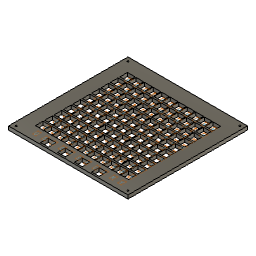
Wordclock (Autodesk Fusion 360 design; units mm, degrees)
Autodesk Fusion 360 part; units mm, degrees
(part 1 of 9)
sketch "Sketch1" plane through (0, 0, 0) normal (0, 0, 1) x (1, 0, 0)
  line L0 (117.5, 117.5) -> (-117.5, 117.5)
  line L1 (-117.5, 117.5) -> (-117.5, -117.5)
  line L2 (-117.5, -117.5) -> (117.5, -117.5)
  line L3 (117.5, -117.5) -> (117.5, 117.5)
  line L4 (117.5, 117.5) -> (-117.5, -117.5) construction
  line L5 (-117.5, 117.5) -> (117.5, -117.5) construction
  circle A0 centre (-110, 110) radius 1.6
  circle A1 centre (110, 110) radius 1.6
  circle A2 centre (-110, -110) radius 1.6
  circle A3 centre (110, -110) radius 1.6
  line L6 (-91.5, 90.5) -> (-76.5, 90.5)
  line L7 (-76.5, 90.5) -> (-76.5, 75.5)
  line L8 (-76.5, 75.5) -> (-91.5, 75.5)
  line L9 (-91.5, 75.5) -> (-91.5, 90.5)
  line L10 (-59.7, 75.5) -> (-74.7, 75.5)
  line L11 (-74.7, 75.5) -> (-74.7, 90.5)
  line L12 (-74.7, 90.5) -> (-59.7, 90.5)
  line L13 (-59.7, 90.5) -> (-59.7, 75.5)
  line L14 (-42.9, 75.5) -> (-57.9, 75.5)
  line L15 (-57.9, 75.5) -> (-57.9, 90.5)
  line L16 (-57.9, 90.5) -> (-42.9, 90.5)
  line L17 (-42.9, 90.5) -> (-42.9, 75.5)
  line L18 (-26.1, 75.5) -> (-41.1, 75.5)
  line L19 (-41.1, 75.5) -> (-41.1, 90.5)
  line L20 (-41.1, 90.5) -> (-26.1, 90.5)
  line L21 (-26.1, 90.5) -> (-26.1, 75.5)
  line L22 (-9.3, 75.5) -> (-24.3, 75.5)
  line L23 (-24.3, 75.5) -> (-24.3, 90.5)
  line L24 (-24.3, 90.5) -> (-9.3, 90.5)
  line L25 (-9.3, 90.5) -> (-9.3, 75.5)
  line L26 (7.5, 75.5) -> (-7.5, 75.5)
  line L27 (-7.5, 75.5) -> (-7.5, 90.5)
  line L28 (-7.5, 90.5) -> (7.5, 90.5)
  line L29 (7.5, 90.5) -> (7.5, 75.5)
  line L30 (24.3, 75.5) -> (9.3, 75.5)
  line L31 (9.3, 75.5) -> (9.3, 90.5)
  line L32 (9.3, 90.5) -> (24.3, 90.5)
  line L33 (24.3, 90.5) -> (24.3, 75.5)
  line L34 (41.1, 75.5) -> (26.1, 75.5)
  line L35 (26.1, 75.5) -> (26.1, 90.5)
  line L36 (26.1, 90.5) -> (41.1, 90.5)
  line L37 (41.1, 90.5) -> (41.1, 75.5)
  line L38 (57.9, 75.5) -> (42.9, 75.5)
  line L39 (42.9, 75.5) -> (42.9, 90.5)
  line L40 (42.9, 90.5) -> (57.9, 90.5)
  line L41 (57.9, 90.5) -> (57.9, 75.5)
  line L42 (74.7, 75.5) -> (59.7, 75.5)
  line L43 (59.7, 75.5) -> (59.7, 90.5)
  line L44 (59.7, 90.5) -> (74.7, 90.5)
  line L45 (74.7, 90.5) -> (74.7, 75.5)
  line L46 (91.5, 75.5) -> (76.5, 75.5)
  line L47 (76.5, 75.5) -> (76.5, 90.5)
  line L48 (76.5, 90.5) -> (91.5, 90.5)
  line L49 (91.5, 90.5) -> (91.5, 75.5)
  line L50 (-76.5, 57.055) -> (-91.5, 57.055)
  line L51 (-91.5, 57.055) -> (-91.5, 72.055)
  line L52 (-91.5, 72.055) -> (-76.5, 72.055)
  line L53 (-76.5, 72.055) -> (-76.5, 57.055)
  line L54 (-59.7, 57.055) -> (-74.7, 57.055)
  line L55 (-74.7, 57.055) -> (-74.7, 72.055)
  line L56 (-74.7, 72.055) -> (-59.7, 72.055)
  line L57 (-59.7, 72.055) -> (-59.7, 57.055)
  line L58 (-42.9, 57.055) -> (-57.9, 57.055)
  line L59 (-57.9, 57.055) -> (-57.9, 72.055)
  line L60 (-57.9, 72.055) -> (-42.9, 72.055)
  line L61 (-42.9, 72.055) -> (-42.9, 57.055)
  line L62 (-26.1, 57.055) -> (-41.1, 57.055)
  line L63 (-41.1, 57.055) -> (-41.1, 72.055)
  line L64 (-41.1, 72.055) -> (-26.1, 72.055)
  line L65 (-26.1, 72.055) -> (-26.1, 57.055)
  line L66 (-9.3, 57.055) -> (-24.3, 57.055)
  line L67 (-24.3, 57.055) -> (-24.3, 72.055)
  line L68 (-24.3, 72.055) -> (-9.3, 72.055)
  line L69 (-9.3, 72.055) -> (-9.3, 57.055)
  line L70 (7.5, 57.055) -> (-7.5, 57.055)
  line L71 (-7.5, 57.055) -> (-7.5, 72.055)
  line L72 (-7.5, 72.055) -> (7.5, 72.055)
  line L73 (7.5, 72.055) -> (7.5, 57.055)
  line L74 (24.3, 57.055) -> (9.3, 57.055)
  line L75 (9.3, 57.055) -> (9.3, 72.055)
  line L76 (9.3, 72.055) -> (24.3, 72.055)
  line L77 (24.3, 72.055) -> (24.3, 57.055)
  line L78 (41.1, 57.055) -> (26.1, 57.055)
  line L79 (26.1, 57.055) -> (26.1, 72.055)
  line L80 (26.1, 72.055) -> (41.1, 72.055)
  line L81 (41.1, 72.055) -> (41.1, 57.055)
  line L82 (57.9, 57.055) -> (42.9, 57.055)
  line L83 (42.9, 57.055) -> (42.9, 72.055)
  line L84 (42.9, 72.055) -> (57.9, 72.055)
  line L85 (57.9, 72.055) -> (57.9, 57.055)
  line L86 (74.7, 57.055) -> (59.7, 57.055)
  line L87 (59.7, 57.055) -> (59.7, 72.055)
  line L88 (59.7, 72.055) -> (74.7, 72.055)
  line L89 (74.7, 72.055) -> (74.7, 57.055)
  line L90 (91.5, 57.055) -> (76.5, 57.055)
  line L91 (76.5, 57.055) -> (76.5, 72.055)
  line L92 (76.5, 72.055) -> (91.5, 72.055)
  line L93 (91.5, 72.055) -> (91.5, 57.055)
  line L94 (-76.5, 38.61) -> (-91.5, 38.61)
  line L95 (-91.5, 38.61) -> (-91.5, 53.61)
  line L96 (-91.5, 53.61) -> (-76.5, 53.61)
  line L97 (-76.5, 53.61) -> (-76.5, 38.61)
  line L98 (-59.7, 38.61) -> (-74.7, 38.61)
  line L99 (-74.7, 38.61) -> (-74.7, 53.61)
  line L100 (-74.7, 53.61) -> (-59.7, 53.61)
  line L101 (-59.7, 53.61) -> (-59.7, 38.61)
  line L102 (-42.9, 38.61) -> (-57.9, 38.61)
  line L103 (-57.9, 38.61) -> (-57.9, 53.61)
  line L104 (-57.9, 53.61) -> (-42.9, 53.61)
  line L105 (-42.9, 53.61) -> (-42.9, 38.61)
  line L106 (-26.1, 38.61) -> (-41.1, 38.61)
  line L107 (-41.1, 38.61) -> (-41.1, 53.61)
  line L108 (-41.1, 53.61) -> (-26.1, 53.61)
  line L109 (-26.1, 53.61) -> (-26.1, 38.61)
  line L110 (-9.3, 38.61) -> (-24.3, 38.61)
  line L111 (-24.3, 38.61) -> (-24.3, 53.61)
  line L112 (-24.3, 53.61) -> (-9.3, 53.61)
  line L113 (-9.3, 53.61) -> (-9.3, 38.61)
  line L114 (7.5, 38.61) -> (-7.5, 38.61)
  line L115 (-7.5, 38.61) -> (-7.5, 53.61)
  line L116 (-7.5, 53.61) -> (7.5, 53.61)
  line L117 (7.5, 53.61) -> (7.5, 38.61)
  line L118 (24.3, 38.61) -> (9.3, 38.61)
  line L119 (9.3, 38.61) -> (9.3, 53.61)
  line L120 (9.3, 53.61) -> (24.3, 53.61)
  line L121 (24.3, 53.61) -> (24.3, 38.61)
  line L122 (41.1, 38.61) -> (26.1, 38.61)
  line L123 (26.1, 38.61) -> (26.1, 53.61)
  line L124 (26.1, 53.61) -> (41.1, 53.61)
  line L125 (41.1, 53.61) -> (41.1, 38.61)
  line L126 (57.9, 38.61) -> (42.9, 38.61)
  line L127 (42.9, 38.61) -> (42.9, 53.61)
  line L128 (42.9, 53.61) -> (57.9, 53.61)
  line L129 (57.9, 53.61) -> (57.9, 38.61)
  line L130 (74.7, 38.61) -> (59.7, 38.61)
  line L131 (59.7, 38.61) -> (59.7, 53.61)
  line L132 (59.7, 53.61) -> (74.7, 53.61)
  line L133 (74.7, 53.61) -> (74.7, 38.61)
  line L134 (91.5, 38.61) -> (76.5, 38.61)
  line L135 (76.5, 38.61) -> (76.5, 53.61)
  line L136 (76.5, 53.61) -> (91.5, 53.61)
  line L137 (91.5, 53.61) -> (91.5, 38.61)
  line L138 (-76.5, 20.165) -> (-91.5, 20.165)
  line L139 (-91.5, 20.165) -> (-91.5, 35.165)
  line L140 (-91.5, 35.165) -> (-76.5, 35.165)
  line L141 (-76.5, 35.165) -> (-76.5, 20.165)
  line L142 (-59.7, 20.165) -> (-74.7, 20.165)
  line L143 (-74.7, 20.165) -> (-74.7, 35.165)
  line L144 (-74.7, 35.165) -> (-59.7, 35.165)
  line L145 (-59.7, 35.165) -> (-59.7, 20.165)
  line L146 (-42.9, 20.165) -> (-57.9, 20.165)
  line L147 (-57.9, 20.165) -> (-57.9, 35.165)
  line L148 (-57.9, 35.165) -> (-42.9, 35.165)
  line L149 (-42.9, 35.165) -> (-42.9, 20.165)
  line L150 (-26.1, 20.165) -> (-41.1, 20.165)
  line L151 (-41.1, 20.165) -> (-41.1, 35.165)
  line L152 (-41.1, 35.165) -> (-26.1, 35.165)
  line L153 (-26.1, 35.165) -> (-26.1, 20.165)
  line L154 (-9.3, 20.165) -> (-24.3, 20.165)
  line L155 (-24.3, 20.165) -> (-24.3, 35.165)
  line L156 (-24.3, 35.165) -> (-9.3, 35.165)
  line L157 (-9.3, 35.165) -> (-9.3, 20.165)
  line L158 (7.5, 20.165) -> (-7.5, 20.165)
  line L159 (-7.5, 20.165) -> (-7.5, 35.165)
  line L160 (-7.5, 35.165) -> (7.5, 35.165)
  line L161 (7.5, 35.165) -> (7.5, 20.165)
  line L162 (24.3, 20.165) -> (9.3, 20.165)
  line L163 (9.3, 20.165) -> (9.3, 35.165)
  line L164 (9.3, 35.165) -> (24.3, 35.165)
  line L165 (24.3, 35.165) -> (24.3, 20.165)
  line L166 (41.1, 20.165) -> (26.1, 20.165)
  line L167 (26.1, 20.165) -> (26.1, 35.165)
  line L168 (26.1, 35.165) -> (41.1, 35.165)
  line L169 (41.1, 35.165) -> (41.1, 20.165)
  line L170 (57.9, 20.165) -> (42.9, 20.165)
  line L171 (42.9, 20.165) -> (42.9, 35.165)
  line L172 (42.9, 35.165) -> (57.9, 35.165)
  line L173 (57.9, 35.165) -> (57.9, 20.165)
  line L174 (74.7, 20.165) -> (59.7, 20.165)
  line L175 (59.7, 20.165) -> (59.7, 35.165)
  line L176 (59.7, 35.165) -> (74.7, 35.165)
  line L177 (74.7, 35.165) -> (74.7, 20.165)
  line L178 (91.5, 20.165) -> (76.5, 20.165)
  line L179 (76.5, 20.165) -> (76.5, 35.165)
  line L180 (76.5, 35.165) -> (91.5, 35.165)
  line L181 (91.5, 35.165) -> (91.5, 20.165)
  line L182 (-76.5, 1.72) -> (-91.5, 1.72)
  line L183 (-91.5, 1.72) -> (-91.5, 16.72)
  line L184 (-91.5, 16.72) -> (-76.5, 16.72)
  line L185 (-76.5, 16.72) -> (-76.5, 1.72)
  line L186 (-59.7, 1.72) -> (-74.7, 1.72)
  line L187 (-74.7, 1.72) -> (-74.7, 16.72)
  line L188 (-74.7, 16.72) -> (-59.7, 16.72)
  line L189 (-59.7, 16.72) -> (-59.7, 1.72)
  line L190 (-42.9, 1.72) -> (-57.9, 1.72)
  line L191 (-57.9, 1.72) -> (-57.9, 16.72)
  line L192 (-57.9, 16.72) -> (-42.9, 16.72)
  line L193 (-42.9, 16.72) -> (-42.9, 1.72)
  line L194 (-26.1, 1.72) -> (-41.1, 1.72)
  line L195 (-41.1, 1.72) -> (-41.1, 16.72)
  line L196 (-41.1, 16.72) -> (-26.1, 16.72)
  line L197 (-26.1, 16.72) -> (-26.1, 1.72)
  line L198 (-9.3, 1.72) -> (-24.3, 1.72)
  line L199 (-24.3, 1.72) -> (-24.3, 16.72)
  line L200 (-24.3, 16.72) -> (-9.3, 16.72)
  line L201 (-9.3, 16.72) -> (-9.3, 1.72)
  line L202 (7.5, 1.72) -> (-7.5, 1.72)
  line L203 (-7.5, 1.72) -> (-7.5, 16.72)
  line L204 (-7.5, 16.72) -> (7.5, 16.72)
  line L205 (7.5, 16.72) -> (7.5, 1.72)
  line L206 (24.3, 1.72) -> (9.3, 1.72)
  line L207 (9.3, 1.72) -> (9.3, 16.72)
  line L208 (9.3, 16.72) -> (24.3, 16.72)
  line L209 (24.3, 16.72) -> (24.3, 1.72)
  line L210 (41.1, 1.72) -> (26.1, 1.72)
  line L211 (26.1, 1.72) -> (26.1, 16.72)
  line L212 (26.1, 16.72) -> (41.1, 16.72)
  line L213 (41.1, 16.72) -> (41.1, 1.72)
  line L214 (57.9, 1.72) -> (42.9, 1.72)
  line L215 (42.9, 1.72) -> (42.9, 16.72)
  line L216 (42.9, 16.72) -> (57.9, 16.72)
  line L217 (57.9, 16.72) -> (57.9, 1.72)
  line L218 (74.7, 1.72) -> (59.7, 1.72)
  line L219 (59.7, 1.72) -> (59.7, 16.72)
  line L220 (59.7, 16.72) -> (74.7, 16.72)
  line L221 (74.7, 16.72) -> (74.7, 1.72)
  line L222 (91.5, 1.72) -> (76.5, 1.72)
  line L223 (76.5, 1.72) -> (76.5, 16.72)
  line L224 (76.5, 16.72) -> (91.5, 16.72)
  line L225 (91.5, 16.72) -> (91.5, 1.72)
  line L226 (-76.5, -16.725) -> (-91.5, -16.725)
  line L227 (-91.5, -16.725) -> (-91.5, -1.725)
  line L228 (-91.5, -1.725) -> (-76.5, -1.725)
  line L229 (-76.5, -1.725) -> (-76.5, -16.725)
  line L230 (-59.7, -16.725) -> (-74.7, -16.725)
  line L231 (-74.7, -16.725) -> (-74.7, -1.725)
  line L232 (-74.7, -1.725) -> (-59.7, -1.725)
  line L233 (-59.7, -1.725) -> (-59.7, -16.725)
  line L234 (-42.9, -16.725) -> (-57.9, -16.725)
  line L235 (-57.9, -16.725) -> (-57.9, -1.725)
  line L236 (-57.9, -1.725) -> (-42.9, -1.725)
  line L237 (-42.9, -1.725) -> (-42.9, -16.725)
  line L238 (-26.1, -16.725) -> (-41.1, -16.725)
  line L239 (-41.1, -16.725) -> (-41.1, -1.725)
  line L240 (-41.1, -1.725) -> (-26.1, -1.725)
  line L241 (-26.1, -1.725) -> (-26.1, -16.725)
  line L242 (-9.3, -16.725) -> (-24.3, -16.725)
  line L243 (-24.3, -16.725) -> (-24.3, -1.725)
  line L244 (-24.3, -1.725) -> (-9.3, -1.725)
  line L245 (-9.3, -1.725) -> (-9.3, -16.725)
  line L246 (7.5, -16.725) -> (-7.5, -16.725)
  line L247 (-7.5, -16.725) -> (-7.5, -1.725)
  line L248 (-7.5, -1.725) -> (7.5, -1.725)
  line L249 (7.5, -1.725) -> (7.5, -16.725)
  line L250 (24.3, -16.725) -> (9.3, -16.725)
  line L251 (9.3, -16.725) -> (9.3, -1.725)
  line L252 (9.3, -1.725) -> (24.3, -1.725)
  line L253 (24.3, -1.725) -> (24.3, -16.725)
  line L254 (41.1, -16.725) -> (26.1, -16.725)
  line L255 (26.1, -16.725) -> (26.1, -1.725)
  line L256 (26.1, -1.725) -> (41.1, -1.725)
  line L257 (41.1, -1.725) -> (41.1, -16.725)
  line L258 (57.9, -16.725) -> (42.9, -16.725)
  line L259 (42.9, -16.725) -> (42.9, -1.725)
  line L260 (42.9, -1.725) -> (57.9, -1.725)
  line L261 (57.9, -1.725) -> (57.9, -16.725)
  line L262 (74.7, -16.725) -> (59.7, -16.725)
  line L263 (59.7, -16.725) -> (59.7, -1.725)
  line L264 (59.7, -1.725) -> (74.7, -1.725)
  line L265 (74.7, -1.725) -> (74.7, -16.725)
  line L266 (91.5, -16.725) -> (76.5, -16.725)
  line L267 (76.5, -16.725) -> (76.5, -1.725)
  line L268 (76.5, -1.725) -> (91.5, -1.725)
  line L269 (91.5, -1.725) -> (91.5, -16.725)
  line L270 (-76.5, -35.17) -> (-91.5, -35.17)
  line L271 (-91.5, -35.17) -> (-91.5, -20.17)
  line L272 (-91.5, -20.17) -> (-76.5, -20.17)
  line L273 (-76.5, -20.17) -> (-76.5, -35.17)
  line L274 (-59.7, -35.17) -> (-74.7, -35.17)
  line L275 (-74.7, -35.17) -> (-74.7, -20.17)
  line L276 (-74.7, -20.17) -> (-59.7, -20.17)
  line L277 (-59.7, -20.17) -> (-59.7, -35.17)
  line L278 (-42.9, -35.17) -> (-57.9, -35.17)
  line L279 (-57.9, -35.17) -> (-57.9, -20.17)
  line L280 (-57.9, -20.17) -> (-42.9, -20.17)
  line L281 (-42.9, -20.17) -> (-42.9, -35.17)
  line L282 (-26.1, -35.17) -> (-41.1, -35.17)
  line L283 (-41.1, -35.17) -> (-41.1, -20.17)
  line L284 (-41.1, -20.17) -> (-26.1, -20.17)
  line L285 (-26.1, -20.17) -> (-26.1, -35.17)
  line L286 (-9.3, -35.17) -> (-24.3, -35.17)
  line L287 (-24.3, -35.17) -> (-24.3, -20.17)
  line L288 (-24.3, -20.17) -> (-9.3, -20.17)
  line L289 (-9.3, -20.17) -> (-9.3, -35.17)
  line L290 (7.5, -35.17) -> (-7.5, -35.17)
  line L291 (-7.5, -35.17) -> (-7.5, -20.17)
  line L292 (-7.5, -20.17) -> (7.5, -20.17)
  line L293 (7.5, -20.17) -> (7.5, -35.17)
  line L294 (24.3, -35.17) -> (9.3, -35.17)
  line L295 (9.3, -35.17) -> (9.3, -20.17)
  line L296 (9.3, -20.17) -> (24.3, -20.17)
  line L297 (24.3, -20.17) -> (24.3, -35.17)
  line L298 (41.1, -35.17) -> (26.1, -35.17)
  line L299 (26.1, -35.17) -> (26.1, -20.17)
  line L300 (26.1, -20.17) -> (41.1, -20.17)
  line L301 (41.1, -20.17) -> (41.1, -35.17)
  line L302 (57.9, -35.17) -> (42.9, -35.17)
  line L303 (42.9, -35.17) -> (42.9, -20.17)
  line L304 (42.9, -20.17) -> (57.9, -20.17)
  line L305 (57.9, -20.17) -> (57.9, -35.17)
  line L306 (74.7, -35.17) -> (59.7, -35.17)
  line L307 (59.7, -35.17) -> (59.7, -20.17)
  line L308 (59.7, -20.17) -> (74.7, -20.17)
  line L309 (74.7, -20.17) -> (74.7, -35.17)
  line L310 (91.5, -35.17) -> (76.5, -35.17)
  line L311 (76.5, -35.17) -> (76.5, -20.17)
  line L312 (76.5, -20.17) -> (91.5, -20.17)
  line L313 (91.5, -20.17) -> (91.5, -35.17)
  line L314 (-76.5, -53.615) -> (-91.5, -53.615)
  line L315 (-91.5, -53.615) -> (-91.5, -38.615)
  line L316 (-91.5, -38.615) -> (-76.5, -38.615)
  line L317 (-76.5, -38.615) -> (-76.5, -53.615)
  line L318 (-59.7, -53.615) -> (-74.7, -53.615)
  line L319 (-74.7, -53.615) -> (-74.7, -38.615)
  line L320 (-74.7, -38.615) -> (-59.7, -38.615)
  line L321 (-59.7, -38.615) -> (-59.7, -53.615)
  line L322 (-42.9, -53.615) -> (-57.9, -53.615)
  line L323 (-57.9, -53.615) -> (-57.9, -38.615)
  line L324 (-57.9, -38.615) -> (-42.9, -38.615)
  line L325 (-42.9, -38.615) -> (-42.9, -53.615)
  line L326 (-26.1, -53.615) -> (-41.1, -53.615)
  line L327 (-41.1, -53.615) -> (-41.1, -38.615)
  line L328 (-41.1, -38.615) -> (-26.1, -38.615)
  line L329 (-26.1, -38.615) -> (-26.1, -53.615)
  line L330 (-9.3, -53.615) -> (-24.3, -53.615)
  line L331 (-24.3, -53.615) -> (-24.3, -38.615)
  line L332 (-24.3, -38.615) -> (-9.3, -38.615)
  line L333 (-9.3, -38.615) -> (-9.3, -53.615)
  line L334 (7.5, -53.615) -> (-7.5, -53.615)
  line L335 (-7.5, -53.615) -> (-7.5, -38.615)
  line L336 (-7.5, -38.615) -> (7.5, -38.615)
  line L337 (7.5, -38.615) -> (7.5, -53.615)
  line L338 (24.3, -53.615) -> (9.3, -53.615)
  line L339 (9.3, -53.615) -> (9.3, -38.615)
  line L340 (9.3, -38.615) -> (24.3, -38.615)
  line L341 (24.3, -38.615) -> (24.3, -53.615)
  line L342 (41.1, -53.615) -> (26.1, -53.615)
  line L343 (26.1, -53.615) -> (26.1, -38.615)
  line L344 (26.1, -38.615) -> (41.1, -38.615)
  line L345 (41.1, -38.615) -> (41.1, -53.615)
  line L346 (57.9, -53.615) -> (42.9, -53.615)
  line L347 (42.9, -53.615) -> (42.9, -38.615)
  line L348 (42.9, -38.615) -> (57.9, -38.615)
  line L349 (57.9, -38.615) -> (57.9, -53.615)
  line L350 (74.7, -53.615) -> (59.7, -53.615)
  line L351 (59.7, -53.615) -> (59.7, -38.615)
  line L352 (59.7, -38.615) -> (74.7, -38.615)
  line L353 (74.7, -38.615) -> (74.7, -53.615)
  line L354 (91.5, -53.615) -> (76.5, -53.615)
  line L355 (76.5, -53.615) -> (76.5, -38.615)
  line L356 (76.5, -38.615) -> (91.5, -38.615)
  line L357 (91.5, -38.615) -> (91.5, -53.615)
  line L358 (-76.5, -72.06) -> (-91.5, -72.06)
  line L359 (-91.5, -72.06) -> (-91.5, -57.06)
  line L360 (-91.5, -57.06) -> (-76.5, -57.06)
  line L361 (-76.5, -57.06) -> (-76.5, -72.06)
  line L362 (-59.7, -72.06) -> (-74.7, -72.06)
  line L363 (-74.7, -72.06) -> (-74.7, -57.06)
  line L364 (-74.7, -57.06) -> (-59.7, -57.06)
  line L365 (-59.7, -57.06) -> (-59.7, -72.06)
  line L366 (-42.9, -72.06) -> (-57.9, -72.06)
  line L367 (-57.9, -72.06) -> (-57.9, -57.06)
  line L368 (-57.9, -57.06) -> (-42.9, -57.06)
  line L369 (-42.9, -57.06) -> (-42.9, -72.06)
  line L370 (-26.1, -72.06) -> (-41.1, -72.06)
  line L371 (-41.1, -72.06) -> (-41.1, -57.06)
  line L372 (-41.1, -57.06) -> (-26.1, -57.06)
  line L373 (-26.1, -57.06) -> (-26.1, -72.06)
  line L374 (-9.3, -72.06) -> (-24.3, -72.06)
  line L375 (-24.3, -72.06) -> (-24.3, -57.06)
  line L376 (-24.3, -57.06) -> (-9.3, -57.06)
  line L377 (-9.3, -57.06) -> (-9.3, -72.06)
  line L378 (7.5, -72.06) -> (-7.5, -72.06)
  line L379 (-7.5, -72.06) -> (-7.5, -57.06)
  line L380 (-7.5, -57.06) -> (7.5, -57.06)
  line L381 (7.5, -57.06) -> (7.5, -72.06)
  line L382 (24.3, -72.06) -> (9.3, -72.06)
  line L383 (9.3, -72.06) -> (9.3, -57.06)
  line L384 (9.3, -57.06) -> (24.3, -57.06)
  line L385 (24.3, -57.06) -> (24.3, -72.06)
  line L386 (41.1, -72.06) -> (26.1, -72.06)
  line L387 (26.1, -72.06) -> (26.1, -57.06)
  line L388 (26.1, -57.06) -> (41.1, -57.06)
  line L389 (41.1, -57.06) -> (41.1, -72.06)
  line L390 (57.9, -72.06) -> (42.9, -72.06)
  line L391 (42.9, -72.06) -> (42.9, -57.06)
  line L392 (42.9, -57.06) -> (57.9, -57.06)
  line L393 (57.9, -57.06) -> (57.9, -72.06)
  line L394 (74.7, -72.06) -> (59.7, -72.06)
  line L395 (59.7, -72.06) -> (59.7, -57.06)
  line L396 (59.7, -57.06) -> (74.7, -57.06)
  line L397 (74.7, -57.06) -> (74.7, -72.06)
  line L398 (91.5, -72.06) -> (76.5, -72.06)
  line L399 (76.5, -72.06) -> (76.5, -57.06)
  line L400 (76.5, -57.06) -> (91.5, -57.06)
  line L401 (91.5, -57.06) -> (91.5, -72.06)
  line L402 (-76.5, -90.505) -> (-91.5, -90.505)
  line L403 (-91.5, -90.505) -> (-91.5, -75.505)
  line L404 (-91.5, -75.505) -> (-76.5, -75.505)
  line L405 (-76.5, -75.505) -> (-76.5, -90.505)
  line L406 (-59.7, -90.505) -> (-74.7, -90.505)
  line L407 (-74.7, -90.505) -> (-74.7, -75.505)
  line L408 (-74.7, -75.505) -> (-59.7, -75.505)
  line L409 (-59.7, -75.505) -> (-59.7, -90.505)
  line L410 (-42.9, -90.505) -> (-57.9, -90.505)
  line L411 (-57.9, -90.505) -> (-57.9, -75.505)
  line L412 (-57.9, -75.505) -> (-42.9, -75.505)
  line L413 (-42.9, -75.505) -> (-42.9, -90.505)
  line L414 (-26.1, -90.505) -> (-41.1, -90.505)
  line L415 (-41.1, -90.505) -> (-41.1, -75.505)
  line L416 (-41.1, -75.505) -> (-26.1, -75.505)
  line L417 (-26.1, -75.505) -> (-26.1, -90.505)
  line L418 (-9.3, -90.505) -> (-24.3, -90.505)
  line L419 (-24.3, -90.505) -> (-24.3, -75.505)
  line L420 (-24.3, -75.505) -> (-9.3, -75.505)
  line L421 (-9.3, -75.505) -> (-9.3, -90.505)
  line L422 (7.5, -90.505) -> (-7.5, -90.505)
  line L423 (-7.5, -90.505) -> (-7.5, -75.505)
  line L424 (-7.5, -75.505) -> (7.5, -75.505)
  line L425 (7.5, -75.505) -> (7.5, -90.505)
  line L426 (24.3, -90.505) -> (9.3, -90.505)
  line L427 (9.3, -90.505) -> (9.3, -75.505)
  line L428 (9.3, -75.505) -> (24.3, -75.505)
  line L429 (24.3, -75.505) -> (24.3, -90.505)
  line L430 (41.1, -90.505) -> (26.1, -90.505)
  line L431 (26.1, -90.505) -> (26.1, -75.505)
  line L432 (26.1, -75.505) -> (41.1, -75.505)
  line L433 (41.1, -75.505) -> (41.1, -90.505)
  line L434 (57.9, -90.505) -> (42.9, -90.505)
  line L435 (42.9, -90.505) -> (42.9, -75.505)
  line L436 (42.9, -75.505) -> (57.9, -75.505)
  line L437 (57.9, -75.505) -> (57.9, -90.505)
  line L438 (74.7, -90.505) -> (59.7, -90.505)
  line L439 (59.7, -90.505) -> (59.7, -75.505)
  line L440 (59.7, -75.505) -> (74.7, -75.505)
  line L441 (74.7, -75.505) -> (74.7, -90.505)
  line L442 (91.5, -90.505) -> (76.5, -90.505)
  line L443 (76.5, -90.505) -> (76.5, -75.505)
  line L444 (76.5, -75.505) -> (91.5, -75.505)
  line L445 (91.5, -75.505) -> (91.5, -90.505)
  line L446 (-57.5, -99.3) -> (-42.5, -99.3)
  line L447 (-42.5, -99.3) -> (-42.5, -114.3)
  line L448 (-42.5, -114.3) -> (-57.5, -114.3)
  line L449 (-57.5, -114.3) -> (-57.5, -99.3)
  line L450 (-24.175, -114.3) -> (-24.175, -99.3)
  line L451 (-24.175, -99.3) -> (-9.175, -99.3)
  line L452 (-9.175, -114.3) -> (-24.175, -114.3)
  line L453 (-9.175, -99.3) -> (-9.175, -114.3)
  line L454 (9.15, -114.3) -> (9.15, -99.3)
  line L455 (9.15, -99.3) -> (24.15, -99.3)
  line L456 (24.15, -114.3) -> (9.15, -114.3)
  line L457 (24.15, -99.3) -> (24.15, -114.3)
  line L458 (42.475, -114.3) -> (42.475, -99.3)
  line L459 (42.475, -99.3) -> (57.475, -99.3)
  line L460 (57.475, -114.3) -> (42.475, -114.3)
  line L461 (57.475, -99.3) -> (57.475, -114.3)
  dimension "d1" = 235
  dimension "d2" = 235
  dimension "d3" = 3.2
  dimension "d4" = 7.5
  dimension "d5" = 7.5
  dimension "d8" = 220
  dimension "d9" = -220
  dimension "d10" = 15
  dimension "d11" = 15
  dimension "d12" = 26
  dimension "d13" = 27
  dimension "d16" = 16.8
  dimension "d17" = -18.445
  dimension "d18" = 15
  dimension "d19" = 15
  dimension "d20" = 60
  dimension "d21" = 3.2
  dimension "d24" = 33.325
  dimension "d25" = 0
  constraint horizontal L0
  constraint perpendicular L0 L1
  constraint parallel L0 L2
  constraint parallel L1 L3
  constraint coincident L4 origin
  constraint coincident L5 origin
  constraint horizontal L6
  constraint vertical L7
  constraint horizontal L8
  constraint vertical L9
  constraint horizontal L446
  constraint vertical L447
  constraint horizontal L448
  constraint vertical L449
  measures "d1" distance of L1.end L2.end
  measures "d2" distance of L0.end L1.end
  measures "d3" diameter of A0
  measures "d4" distance of L1 A0.centre
  measures "d5" distance of L0 A0.centre
  measures "d10" distance of L7 L9
  measures "d11" distance of L6 L8
  measures "d12" distance of L1 L9
  measures "d13" distance of L0 L6
  measures "d18" distance of L447 L449
  measures "d19" distance of L446 L448
  measures "d20" distance of L1 L449
  measures "d21" distance of L2 L448
extrude "Extrude1" add sketch "Sketch1" along normal blind 5
sketch "Sketch2" plane through (0, 0, 0) normal (0, 0, 1) x (1, 0, 0)
  line L0 (-85.5, 85.3) -> (-80.5, 85.3)
  line L1 (-80.5, 85.3) -> (-80.5, 80.3)
  line L2 (-80.5, 80.3) -> (-85.5, 80.3)
  line L3 (-85.5, 80.3) -> (-85.5, 85.3)
  line L4 (117.5, 117.5) -> (-117.5, 117.5)
  line L5 (-117.5, 117.5) -> (-117.5, -117.5)
  line L6 (-69.02, 80.3) -> (-69.02, 85.3)
  line L7 (-69.02, 85.3) -> (-64.02, 85.3)
  line L8 (-64.02, 85.3) -> (-64.02, 80.3)
  line L9 (-64.02, 80.3) -> (-69.02, 80.3)
  line L10 (-52.54, 80.3) -> (-52.54, 85.3)
  line L11 (-52.54, 85.3) -> (-47.54, 85.3)
  line L12 (-47.54, 85.3) -> (-47.54, 80.3)
  line L13 (-47.54, 80.3) -> (-52.54, 80.3)
  line L14 (-36.06, 80.3) -> (-36.06, 85.3)
  line L15 (-36.06, 85.3) -> (-31.06, 85.3)
  line L16 (-31.06, 85.3) -> (-31.06, 80.3)
  line L17 (-31.06, 80.3) -> (-36.06, 80.3)
  line L18 (-19.58, 80.3) -> (-19.58, 85.3)
  line L19 (-19.58, 85.3) -> (-14.58, 85.3)
  line L20 (-14.58, 85.3) -> (-14.58, 80.3)
  line L21 (-14.58, 80.3) -> (-19.58, 80.3)
  line L22 (-3.1, 80.3) -> (-3.1, 85.3)
  line L23 (-3.1, 85.3) -> (1.9, 85.3)
  line L24 (1.9, 85.3) -> (1.9, 80.3)
  line L25 (1.9, 80.3) -> (-3.1, 80.3)
  line L26 (13.38, 80.3) -> (13.38, 85.3)
  line L27 (13.38, 85.3) -> (18.38, 85.3)
  line L28 (18.38, 85.3) -> (18.38, 80.3)
  line L29 (18.38, 80.3) -> (13.38, 80.3)
  line L30 (29.86, 80.3) -> (29.86, 85.3)
  line L31 (29.86, 85.3) -> (34.86, 85.3)
  line L32 (34.86, 85.3) -> (34.86, 80.3)
  line L33 (34.86, 80.3) -> (29.86, 80.3)
  line L34 (46.34, 80.3) -> (46.34, 85.3)
  line L35 (46.34, 85.3) -> (51.34, 85.3)
  line L36 (51.34, 85.3) -> (51.34, 80.3)
  line L37 (51.34, 80.3) -> (46.34, 80.3)
  line L38 (62.82, 80.3) -> (62.82, 85.3)
  line L39 (62.82, 85.3) -> (67.82, 85.3)
  line L40 (67.82, 85.3) -> (67.82, 80.3)
  line L41 (67.82, 80.3) -> (62.82, 80.3)
  line L42 (79.3, 80.3) -> (79.3, 85.3)
  line L43 (79.3, 85.3) -> (84.3, 85.3)
  line L44 (84.3, 85.3) -> (84.3, 80.3)
  line L45 (84.3, 80.3) -> (79.3, 80.3)
  line L46 (-85.5, 61.92) -> (-85.5, 66.92)
  line L47 (-85.5, 66.92) -> (-80.5, 66.92)
  line L48 (-80.5, 66.92) -> (-80.5, 61.92)
  line L49 (-80.5, 61.92) -> (-85.5, 61.92)
  line L50 (-69.02, 61.92) -> (-69.02, 66.92)
  line L51 (-69.02, 66.92) -> (-64.02, 66.92)
  line L52 (-64.02, 66.92) -> (-64.02, 61.92)
  line L53 (-64.02, 61.92) -> (-69.02, 61.92)
  line L54 (-52.54, 61.92) -> (-52.54, 66.92)
  line L55 (-52.54, 66.92) -> (-47.54, 66.92)
  line L56 (-47.54, 66.92) -> (-47.54, 61.92)
  line L57 (-47.54, 61.92) -> (-52.54, 61.92)
  line L58 (-36.06, 61.92) -> (-36.06, 66.92)
  line L59 (-36.06, 66.92) -> (-31.06, 66.92)
  line L60 (-31.06, 66.92) -> (-31.06, 61.92)
  line L61 (-31.06, 61.92) -> (-36.06, 61.92)
  line L62 (-19.58, 61.92) -> (-19.58, 66.92)
  line L63 (-19.58, 66.92) -> (-14.58, 66.92)
  line L64 (-14.58, 66.92) -> (-14.58, 61.92)
  line L65 (-14.58, 61.92) -> (-19.58, 61.92)
  line L66 (-3.1, 61.92) -> (-3.1, 66.92)
  line L67 (-3.1, 66.92) -> (1.9, 66.92)
  line L68 (1.9, 66.92) -> (1.9, 61.92)
  line L69 (1.9, 61.92) -> (-3.1, 61.92)
  line L70 (13.38, 61.92) -> (13.38, 66.92)
  line L71 (13.38, 66.92) -> (18.38, 66.92)
  line L72 (18.38, 66.92) -> (18.38, 61.92)
  line L73 (18.38, 61.92) -> (13.38, 61.92)
  line L74 (29.86, 61.92) -> (29.86, 66.92)
  line L75 (29.86, 66.92) -> (34.86, 66.92)
  line L76 (34.86, 66.92) -> (34.86, 61.92)
  line L77 (34.86, 61.92) -> (29.86, 61.92)
  line L78 (46.34, 61.92) -> (46.34, 66.92)
  line L79 (46.34, 66.92) -> (51.34, 66.92)
  line L80 (51.34, 66.92) -> (51.34, 61.92)
  line L81 (51.34, 61.92) -> (46.34, 61.92)
  line L82 (62.82, 61.92) -> (62.82, 66.92)
  line L83 (62.82, 66.92) -> (67.82, 66.92)
  line L84 (67.82, 66.92) -> (67.82, 61.92)
  line L85 (67.82, 61.92) -> (62.82, 61.92)
  line L86 (79.3, 61.92) -> (79.3, 66.92)
  line L87 (79.3, 66.92) -> (84.3, 66.92)
  line L88 (84.3, 66.92) -> (84.3, 61.92)
  line L89 (84.3, 61.92) -> (79.3, 61.92)
  line L90 (-85.5, 43.54) -> (-85.5, 48.54)
  line L91 (-85.5, 48.54) -> (-80.5, 48.54)
  line L92 (-80.5, 48.54) -> (-80.5, 43.54)
  line L93 (-80.5, 43.54) -> (-85.5, 43.54)
  line L94 (-69.02, 43.54) -> (-69.02, 48.54)
  line L95 (-69.02, 48.54) -> (-64.02, 48.54)
  line L96 (-64.02, 48.54) -> (-64.02, 43.54)
  line L97 (-64.02, 43.54) -> (-69.02, 43.54)
  line L98 (-52.54, 43.54) -> (-52.54, 48.54)
  line L99 (-52.54, 48.54) -> (-47.54, 48.54)
  line L100 (-47.54, 48.54) -> (-47.54, 43.54)
  line L101 (-47.54, 43.54) -> (-52.54, 43.54)
  line L102 (-36.06, 43.54) -> (-36.06, 48.54)
  line L103 (-36.06, 48.54) -> (-31.06, 48.54)
  line L104 (-31.06, 48.54) -> (-31.06, 43.54)
  line L105 (-31.06, 43.54) -> (-36.06, 43.54)
  line L106 (-19.58, 43.54) -> (-19.58, 48.54)
  line L107 (-19.58, 48.54) -> (-14.58, 48.54)
  line L108 (-14.58, 48.54) -> (-14.58, 43.54)
  line L109 (-14.58, 43.54) -> (-19.58, 43.54)
  line L110 (-3.1, 43.54) -> (-3.1, 48.54)
  line L111 (-3.1, 48.54) -> (1.9, 48.54)
  line L112 (1.9, 48.54) -> (1.9, 43.54)
  line L113 (1.9, 43.54) -> (-3.1, 43.54)
  line L114 (13.38, 43.54) -> (13.38, 48.54)
  line L115 (13.38, 48.54) -> (18.38, 48.54)
  line L116 (18.38, 48.54) -> (18.38, 43.54)
  line L117 (18.38, 43.54) -> (13.38, 43.54)
  line L118 (29.86, 43.54) -> (29.86, 48.54)
  line L119 (29.86, 48.54) -> (34.86, 48.54)
  line L120 (34.86, 48.54) -> (34.86, 43.54)
  line L121 (34.86, 43.54) -> (29.86, 43.54)
  line L122 (46.34, 43.54) -> (46.34, 48.54)
  line L123 (46.34, 48.54) -> (51.34, 48.54)
  line L124 (51.34, 48.54) -> (51.34, 43.54)
  line L125 (51.34, 43.54) -> (46.34, 43.54)
  line L126 (62.82, 43.54) -> (62.82, 48.54)
  line L127 (62.82, 48.54) -> (67.82, 48.54)
  line L128 (67.82, 48.54) -> (67.82, 43.54)
  line L129 (67.82, 43.54) -> (62.82, 43.54)
  line L130 (79.3, 43.54) -> (79.3, 48.54)
  line L131 (79.3, 48.54) -> (84.3, 48.54)
  line L132 (84.3, 48.54) -> (84.3, 43.54)
  line L133 (84.3, 43.54) -> (79.3, 43.54)
  line L134 (-85.5, 25.16) -> (-85.5, 30.16)
  line L135 (-85.5, 30.16) -> (-80.5, 30.16)
  line L136 (-80.5, 30.16) -> (-80.5, 25.16)
  line L137 (-80.5, 25.16) -> (-85.5, 25.16)
  line L138 (-69.02, 25.16) -> (-69.02, 30.16)
  line L139 (-69.02, 30.16) -> (-64.02, 30.16)
  line L140 (-64.02, 30.16) -> (-64.02, 25.16)
  line L141 (-64.02, 25.16) -> (-69.02, 25.16)
  line L142 (-52.54, 25.16) -> (-52.54, 30.16)
  line L143 (-52.54, 30.16) -> (-47.54, 30.16)
  line L144 (-47.54, 30.16) -> (-47.54, 25.16)
  line L145 (-47.54, 25.16) -> (-52.54, 25.16)
  line L146 (-36.06, 25.16) -> (-36.06, 30.16)
  line L147 (-36.06, 30.16) -> (-31.06, 30.16)
  line L148 (-31.06, 30.16) -> (-31.06, 25.16)
  line L149 (-31.06, 25.16) -> (-36.06, 25.16)
  line L150 (-19.58, 25.16) -> (-19.58, 30.16)
  line L151 (-19.58, 30.16) -> (-14.58, 30.16)
  line L152 (-14.58, 30.16) -> (-14.58, 25.16)
  line L153 (-14.58, 25.16) -> (-19.58, 25.16)
  line L154 (-3.1, 25.16) -> (-3.1, 30.16)
  line L155 (-3.1, 30.16) -> (1.9, 30.16)
  line L156 (1.9, 30.16) -> (1.9, 25.16)
  line L157 (1.9, 25.16) -> (-3.1, 25.16)
  line L158 (13.38, 25.16) -> (13.38, 30.16)
  line L159 (13.38, 30.16) -> (18.38, 30.16)
  line L160 (18.38, 30.16) -> (18.38, 25.16)
  line L161 (18.38, 25.16) -> (13.38, 25.16)
  line L162 (29.86, 25.16) -> (29.86, 30.16)
  line L163 (29.86, 30.16) -> (34.86, 30.16)
  line L164 (34.86, 30.16) -> (34.86, 25.16)
  line L165 (34.86, 25.16) -> (29.86, 25.16)
  line L166 (46.34, 25.16) -> (46.34, 30.16)
  line L167 (46.34, 30.16) -> (51.34, 30.16)
  line L168 (51.34, 30.16) -> (51.34, 25.16)
  line L169 (51.34, 25.16) -> (46.34, 25.16)
  line L170 (62.82, 25.16) -> (62.82, 30.16)
  line L171 (62.82, 30.16) -> (67.82, 30.16)
  line L172 (67.82, 30.16) -> (67.82, 25.16)
  line L173 (67.82, 25.16) -> (62.82, 25.16)
  line L174 (79.3, 25.16) -> (79.3, 30.16)
  line L175 (79.3, 30.16) -> (84.3, 30.16)
  line L176 (84.3, 30.16) -> (84.3, 25.16)
  line L177 (84.3, 25.16) -> (79.3, 25.16)
  line L178 (-85.5, 6.78) -> (-85.5, 11.78)
  line L179 (-85.5, 11.78) -> (-80.5, 11.78)
  line L180 (-80.5, 11.78) -> (-80.5, 6.78)
  line L181 (-80.5, 6.78) -> (-85.5, 6.78)
  line L182 (-69.02, 6.78) -> (-69.02, 11.78)
  line L183 (-69.02, 11.78) -> (-64.02, 11.78)
  line L184 (-64.02, 11.78) -> (-64.02, 6.78)
  line L185 (-64.02, 6.78) -> (-69.02, 6.78)
  line L186 (-52.54, 6.78) -> (-52.54, 11.78)
  line L187 (-52.54, 11.78) -> (-47.54, 11.78)
  line L188 (-47.54, 11.78) -> (-47.54, 6.78)
  line L189 (-47.54, 6.78) -> (-52.54, 6.78)
  line L190 (-36.06, 6.78) -> (-36.06, 11.78)
  line L191 (-36.06, 11.78) -> (-31.06, 11.78)
  line L192 (-31.06, 11.78) -> (-31.06, 6.78)
  line L193 (-31.06, 6.78) -> (-36.06, 6.78)
  line L194 (-19.58, 6.78) -> (-19.58, 11.78)
  line L195 (-19.58, 11.78) -> (-14.58, 11.78)
  line L196 (-14.58, 11.78) -> (-14.58, 6.78)
  line L197 (-14.58, 6.78) -> (-19.58, 6.78)
  line L198 (-3.1, 6.78) -> (-3.1, 11.78)
  line L199 (-3.1, 11.78) -> (1.9, 11.78)
  line L200 (1.9, 11.78) -> (1.9, 6.78)
  line L201 (1.9, 6.78) -> (-3.1, 6.78)
  line L202 (13.38, 6.78) -> (13.38, 11.78)
  line L203 (13.38, 11.78) -> (18.38, 11.78)
  line L204 (18.38, 11.78) -> (18.38, 6.78)
  line L205 (18.38, 6.78) -> (13.38, 6.78)
  line L206 (29.86, 6.78) -> (29.86, 11.78)
  line L207 (29.86, 11.78) -> (34.86, 11.78)
  line L208 (34.86, 11.78) -> (34.86, 6.78)
  line L209 (34.86, 6.78) -> (29.86, 6.78)
  line L210 (46.34, 6.78) -> (46.34, 11.78)
  line L211 (46.34, 11.78) -> (51.34, 11.78)
  line L212 (51.34, 11.78) -> (51.34, 6.78)
  line L213 (51.34, 6.78) -> (46.34, 6.78)
  line L214 (62.82, 6.78) -> (62.82, 11.78)
  line L215 (62.82, 11.78) -> (67.82, 11.78)
  line L216 (67.82, 11.78) -> (67.82, 6.78)
  line L217 (67.82, 6.78) -> (62.82, 6.78)
  line L218 (79.3, 6.78) -> (79.3, 11.78)
  line L219 (79.3, 11.78) -> (84.3, 11.78)
  line L220 (84.3, 11.78) -> (84.3, 6.78)
  line L221 (84.3, 6.78) -> (79.3, 6.78)
  line L222 (-85.5, -11.6) -> (-85.5, -6.6)
  line L223 (-85.5, -6.6) -> (-80.5, -6.6)
  line L224 (-80.5, -6.6) -> (-80.5, -11.6)
  line L225 (-80.5, -11.6) -> (-85.5, -11.6)
  line L226 (-69.02, -11.6) -> (-69.02, -6.6)
  line L227 (-69.02, -6.6) -> (-64.02, -6.6)
  line L228 (-64.02, -6.6) -> (-64.02, -11.6)
  line L229 (-64.02, -11.6) -> (-69.02, -11.6)
  line L230 (-52.54, -11.6) -> (-52.54, -6.6)
  line L231 (-52.54, -6.6) -> (-47.54, -6.6)
  line L232 (-47.54, -6.6) -> (-47.54, -11.6)
  line L233 (-47.54, -11.6) -> (-52.54, -11.6)
  line L234 (-36.06, -11.6) -> (-36.06, -6.6)
  line L235 (-36.06, -6.6) -> (-31.06, -6.6)
  line L236 (-31.06, -6.6) -> (-31.06, -11.6)
  line L237 (-31.06, -11.6) -> (-36.06, -11.6)
  line L238 (-19.58, -11.6) -> (-19.58, -6.6)
  line L239 (-19.58, -6.6) -> (-14.58, -6.6)
  line L240 (-14.58, -6.6) -> (-14.58, -11.6)
  line L241 (-14.58, -11.6) -> (-19.58, -11.6)
  line L242 (-3.1, -11.6) -> (-3.1, -6.6)
  line L243 (-3.1, -6.6) -> (1.9, -6.6)
  line L244 (1.9, -6.6) -> (1.9, -11.6)
  line L245 (1.9, -11.6) -> (-3.1, -11.6)
  line L246 (13.38, -11.6) -> (13.38, -6.6)
  line L247 (13.38, -6.6) -> (18.38, -6.6)
  line L248 (18.38, -6.6) -> (18.38, -11.6)
  line L249 (18.38, -11.6) -> (13.38, -11.6)
  line L250 (29.86, -11.6) -> (29.86, -6.6)
  line L251 (29.86, -6.6) -> (34.86, -6.6)
  line L252 (34.86, -6.6) -> (34.86, -11.6)
  line L253 (34.86, -11.6) -> (29.86, -11.6)
  line L254 (46.34, -11.6) -> (46.34, -6.6)
  line L255 (46.34, -6.6) -> (51.34, -6.6)
  line L256 (51.34, -6.6) -> (51.34, -11.6)
  line L257 (51.34, -11.6) -> (46.34, -11.6)
  line L258 (62.82, -11.6) -> (62.82, -6.6)
  line L259 (62.82, -6.6) -> (67.82, -6.6)
  line L260 (67.82, -6.6) -> (67.82, -11.6)
  line L261 (67.82, -11.6) -> (62.82, -11.6)
  line L262 (79.3, -11.6) -> (79.3, -6.6)
  line L263 (79.3, -6.6) -> (84.3, -6.6)
  line L264 (84.3, -6.6) -> (84.3, -11.6)
  line L265 (84.3, -11.6) -> (79.3, -11.6)
  line L266 (-85.5, -29.98) -> (-85.5, -24.98)
  line L267 (-85.5, -24.98) -> (-80.5, -24.98)
  line L268 (-80.5, -24.98) -> (-80.5, -29.98)
  line L269 (-80.5, -29.98) -> (-85.5, -29.98)
  line L270 (-69.02, -29.98) -> (-69.02, -24.98)
  line L271 (-69.02, -24.98) -> (-64.02, -24.98)
  line L272 (-64.02, -24.98) -> (-64.02, -29.98)
  line L273 (-64.02, -29.98) -> (-69.02, -29.98)
  line L274 (-52.54, -29.98) -> (-52.54, -24.98)
  line L275 (-52.54, -24.98) -> (-47.54, -24.98)
  line L276 (-47.54, -24.98) -> (-47.54, -29.98)
  line L277 (-47.54, -29.98) -> (-52.54, -29.98)
  line L278 (-36.06, -29.98) -> (-36.06, -24.98)
  line L279 (-36.06, -24.98) -> (-31.06, -24.98)
  line L280 (-31.06, -24.98) -> (-31.06, -29.98)
  line L281 (-31.06, -29.98) -> (-36.06, -29.98)
  line L282 (-19.58, -29.98) -> (-19.58, -24.98)
  line L283 (-19.58, -24.98) -> (-14.58, -24.98)
  line L284 (-14.58, -24.98) -> (-14.58, -29.98)
  line L285 (-14.58, -29.98) -> (-19.58, -29.98)
  line L286 (-3.1, -29.98) -> (-3.1, -24.98)
  line L287 (-3.1, -24.98) -> (1.9, -24.98)
  line L288 (1.9, -24.98) -> (1.9, -29.98)
  line L289 (1.9, -29.98) -> (-3.1, -29.98)
  line L290 (13.38, -29.98) -> (13.38, -24.98)
  line L291 (13.38, -24.98) -> (18.38, -24.98)
  line L292 (18.38, -24.98) -> (18.38, -29.98)
  line L293 (18.38, -29.98) -> (13.38, -29.98)
  line L294 (29.86, -29.98) -> (29.86, -24.98)
  line L295 (29.86, -24.98) -> (34.86, -24.98)
  line L296 (34.86, -24.98) -> (34.86, -29.98)
  line L297 (34.86, -29.98) -> (29.86, -29.98)
  line L298 (46.34, -29.98) -> (46.34, -24.98)
  line L299 (46.34, -24.98) -> (51.34, -24.98)
  line L300 (51.34, -24.98) -> (51.34, -29.98)
  line L301 (51.34, -29.98) -> (46.34, -29.98)
  line L302 (62.82, -29.98) -> (62.82, -24.98)
  line L303 (62.82, -24.98) -> (67.82, -24.98)
  line L304 (67.82, -24.98) -> (67.82, -29.98)
  line L305 (67.82, -29.98) -> (62.82, -29.98)
  line L306 (79.3, -29.98) -> (79.3, -24.98)
  line L307 (79.3, -24.98) -> (84.3, -24.98)
  line L308 (84.3, -24.98) -> (84.3, -29.98)
  line L309 (84.3, -29.98) -> (79.3, -29.98)
  line L310 (-85.5, -48.36) -> (-85.5, -43.36)
  line L311 (-85.5, -43.36) -> (-80.5, -43.36)
  line L312 (-80.5, -43.36) -> (-80.5, -48.36)
  line L313 (-80.5, -48.36) -> (-85.5, -48.36)
  line L314 (-69.02, -48.36) -> (-69.02, -43.36)
  line L315 (-69.02, -43.36) -> (-64.02, -43.36)
  line L316 (-64.02, -43.36) -> (-64.02, -48.36)
  line L317 (-64.02, -48.36) -> (-69.02, -48.36)
  line L318 (-52.54, -48.36) -> (-52.54, -43.36)
  line L319 (-52.54, -43.36) -> (-47.54, -43.36)
  line L320 (-47.54, -43.36) -> (-47.54, -48.36)
  line L321 (-47.54, -48.36) -> (-52.54, -48.36)
  line L322 (-36.06, -48.36) -> (-36.06, -43.36)
  line L323 (-36.06, -43.36) -> (-31.06, -43.36)
  line L324 (-31.06, -43.36) -> (-31.06, -48.36)
  line L325 (-31.06, -48.36) -> (-36.06, -48.36)
  line L326 (-19.58, -48.36) -> (-19.58, -43.36)
  line L327 (-19.58, -43.36) -> (-14.58, -43.36)
  line L328 (-14.58, -43.36) -> (-14.58, -48.36)
  line L329 (-14.58, -48.36) -> (-19.58, -48.36)
  line L330 (-3.1, -48.36) -> (-3.1, -43.36)
  line L331 (-3.1, -43.36) -> (1.9, -43.36)
  line L332 (1.9, -43.36) -> (1.9, -48.36)
  line L333 (1.9, -48.36) -> (-3.1, -48.36)
  line L334 (13.38, -48.36) -> (13.38, -43.36)
  line L335 (13.38, -43.36) -> (18.38, -43.36)
  line L336 (18.38, -43.36) -> (18.38, -48.36)
  line L337 (18.38, -48.36) -> (13.38, -48.36)
  line L338 (29.86, -48.36) -> (29.86, -43.36)
  line L339 (29.86, -43.36) -> (34.86, -43.36)
  line L340 (34.86, -43.36) -> (34.86, -48.36)
  line L341 (34.86, -48.36) -> (29.86, -48.36)
  line L342 (46.34, -48.36) -> (46.34, -43.36)
  line L343 (46.34, -43.36) -> (51.34, -43.36)
  line L344 (51.34, -43.36) -> (51.34, -48.36)
  line L345 (51.34, -48.36) -> (46.34, -48.36)
  line L346 (62.82, -48.36) -> (62.82, -43.36)
  line L347 (62.82, -43.36) -> (67.82, -43.36)
  line L348 (67.82, -43.36) -> (67.82, -48.36)
  line L349 (67.82, -48.36) -> (62.82, -48.36)
  line L350 (79.3, -48.36) -> (79.3, -43.36)
  line L351 (79.3, -43.36) -> (84.3, -43.36)
  line L352 (84.3, -43.36) -> (84.3, -48.36)
  line L353 (84.3, -48.36) -> (79.3, -48.36)
  line L354 (-85.5, -66.74) -> (-85.5, -61.74)
  line L355 (-85.5, -61.74) -> (-80.5, -61.74)
  line L356 (-80.5, -61.74) -> (-80.5, -66.74)
  line L357 (-80.5, -66.74) -> (-85.5, -66.74)
  line L358 (-69.02, -66.74) -> (-69.02, -61.74)
  line L359 (-69.02, -61.74) -> (-64.02, -61.74)
  line L360 (-64.02, -61.74) -> (-64.02, -66.74)
  line L361 (-64.02, -66.74) -> (-69.02, -66.74)
  line L362 (-52.54, -66.74) -> (-52.54, -61.74)
  line L363 (-52.54, -61.74) -> (-47.54, -61.74)
  line L364 (-47.54, -61.74) -> (-47.54, -66.74)
  line L365 (-47.54, -66.74) -> (-52.54, -66.74)
  line L366 (-36.06, -66.74) -> (-36.06, -61.74)
  line L367 (-36.06, -61.74) -> (-31.06, -61.74)
  line L368 (-31.06, -61.74) -> (-31.06, -66.74)
  line L369 (-31.06, -66.74) -> (-36.06, -66.74)
  line L370 (-19.58, -66.74) -> (-19.58, -61.74)
  line L371 (-19.58, -61.74) -> (-14.58, -61.74)
  line L372 (-14.58, -61.74) -> (-14.58, -66.74)
  line L373 (-14.58, -66.74) -> (-19.58, -66.74)
  line L374 (-3.1, -66.74) -> (-3.1, -61.74)
  line L375 (-3.1, -61.74) -> (1.9, -61.74)
  line L376 (1.9, -61.74) -> (1.9, -66.74)
  line L377 (1.9, -66.74) -> (-3.1, -66.74)
  line L378 (13.38, -66.74) -> (13.38, -61.74)
  line L379 (13.38, -61.74) -> (18.38, -61.74)
  line L380 (18.38, -61.74) -> (18.38, -66.74)
  line L381 (18.38, -66.74) -> (13.38, -66.74)
  line L382 (29.86, -66.74) -> (29.86, -61.74)
  line L383 (29.86, -61.74) -> (34.86, -61.74)
  line L384 (34.86, -61.74) -> (34.86, -66.74)
  line L385 (34.86, -66.74) -> (29.86, -66.74)
  line L386 (46.34, -66.74) -> (46.34, -61.74)
  line L387 (46.34, -61.74) -> (51.34, -61.74)
  line L388 (51.34, -61.74) -> (51.34, -66.74)
  line L389 (51.34, -66.74) -> (46.34, -66.74)
  line L390 (62.82, -66.74) -> (62.82, -61.74)
  line L391 (62.82, -61.74) -> (67.82, -61.74)
  line L392 (67.82, -61.74) -> (67.82, -66.74)
  line L393 (67.82, -66.74) -> (62.82, -66.74)
  line L394 (79.3, -66.74) -> (79.3, -61.74)
  line L395 (79.3, -61.74) -> (84.3, -61.74)
  line L396 (84.3, -61.74) -> (84.3, -66.74)
  line L397 (84.3, -66.74) -> (79.3, -66.74)
  line L398 (-85.5, -85.12) -> (-85.5, -80.12)
  line L399 (-85.5, -80.12) -> (-80.5, -80.12)
  line L400 (-80.5, -80.12) -> (-80.5, -85.12)
  line L401 (-80.5, -85.12) -> (-85.5, -85.12)
  line L402 (-69.02, -85.12) -> (-69.02, -80.12)
  line L403 (-69.02, -80.12) -> (-64.02, -80.12)
  line L404 (-64.02, -80.12) -> (-64.02, -85.12)
  line L405 (-64.02, -85.12) -> (-69.02, -85.12)
  line L406 (-52.54, -85.12) -> (-52.54, -80.12)
  line L407 (-52.54, -80.12) -> (-47.54, -80.12)
  line L408 (-47.54, -80.12) -> (-47.54, -85.12)
  line L409 (-47.54, -85.12) -> (-52.54, -85.12)
  line L410 (-36.06, -85.12) -> (-36.06, -80.12)
  line L411 (-36.06, -80.12) -> (-31.06, -80.12)
  line L412 (-31.06, -80.12) -> (-31.06, -85.12)
  line L413 (-31.06, -85.12) -> (-36.06, -85.12)
  line L414 (-19.58, -85.12) -> (-19.58, -80.12)
  line L415 (-19.58, -80.12) -> (-14.58, -80.12)
  line L416 (-14.58, -80.12) -> (-14.58, -85.12)
  line L417 (-14.58, -85.12) -> (-19.58, -85.12)
  line L418 (-3.1, -85.12) -> (-3.1, -80.12)
  line L419 (-3.1, -80.12) -> (1.9, -80.12)
  line L420 (1.9, -80.12) -> (1.9, -85.12)
  line L421 (1.9, -85.12) -> (-3.1, -85.12)
  line L422 (13.38, -85.12) -> (13.38, -80.12)
  line L423 (13.38, -80.12) -> (18.38, -80.12)
  line L424 (18.38, -80.12) -> (18.38, -85.12)
  line L425 (18.38, -85.12) -> (13.38, -85.12)
  line L426 (29.86, -85.12) -> (29.86, -80.12)
  line L427 (29.86, -80.12) -> (34.86, -80.12)
  line L428 (34.86, -80.12) -> (34.86, -85.12)
  line L429 (34.86, -85.12) -> (29.86, -85.12)
  line L430 (46.34, -85.12) -> (46.34, -80.12)
  line L431 (46.34, -80.12) -> (51.34, -80.12)
  line L432 (51.34, -80.12) -> (51.34, -85.12)
  line L433 (51.34, -85.12) -> (46.34, -85.12)
  line L434 (62.82, -85.12) -> (62.82, -80.12)
  line L435 (62.82, -80.12) -> (67.82, -80.12)
  line L436 (67.82, -80.12) -> (67.82, -85.12)
  line L437 (67.82, -85.12) -> (62.82, -85.12)
  line L438 (79.3, -85.12) -> (79.3, -80.12)
  line L439 (79.3, -80.12) -> (84.3, -80.12)
  line L440 (84.3, -80.12) -> (84.3, -85.12)
  line L441 (84.3, -85.12) -> (79.3, -85.12)
  dimension "d28" = 5
  dimension "d29" = 5
  dimension "d30" = 32.2
  dimension "d31" = 32
  dimension "d34" = 16.48
  dimension "d35" = -18.38
  constraint horizontal L0
  constraint vertical L1
  constraint horizontal L2
  constraint vertical L3
  measures "d28" distance of L0.start L2.end
  measures "d29" distance of L0.start L0.end
  measures "d30" distance of L0 L4
  measures "d31" distance of L3 L5